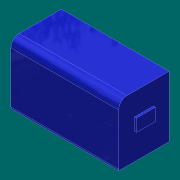
# Autodesk Inventor part: Blue tool box
Saved by Autodesk Inventor 2017 (Build 210142000, 142)
## iProperties
Created: 2018-01-23
Part Number: Blue tool box
Material: Steel
Document SubType Name: Modeling
Designer: Graeme_Van_Dongen
Density: 7.85 g/cm^3
Appearance: Blue - Wall Paint - Glossy
Author: Graeme_Van_Dongen
Autodesk Inventor part; units mm, degrees
ref_plane "YZ Plane" through (0, 0, 0) normal (1, 0, 0) x (0, 1, 0)
ref_plane "XZ Plane" through (0, 0, 0) normal (0, 1, 0) x (-1, 0, 0)
ref_plane "XY Plane" through (0, 0, 0) normal (0, 0, 1) x (1, 0, 0)
sketch "Sketch1" plane through (0, 0, 0) normal (0, 1, 0) x (-1, 0, 0)
  line L0 (330.2, 153.9875) -> (-330.2, 153.9875)
  line L1 (-330.2, 153.9875) -> (-330.2, -153.9875)
  line L2 (-330.2, -153.9875) -> (330.2, -153.9875)
  line L3 (330.2, -153.9875) -> (330.2, 153.9875)
  line L4 (330.2, 153.9875) -> (-330.2, -153.9875) construction
  line L5 (-330.2, 153.9875) -> (330.2, -153.9875) construction
  point P0 (0, 0)
  dimension "d0" = 660.4
  dimension "d1" = 307.975
  constraints: 12 end point, 2 midpoint, 2 parallel, 1 horizontal, 1 perpendicular
  measures "d0" distance of L2.end L1.end
  measures "d1" distance of L1.end L0.end
extrude "Extrusion1" add sketch "Sketch1" along normal blind 374.65
sketch "Sketch4" plane through (330.2, 0, 153.9875) normal (1, 0, 0) x (0, 0, -1)
  line L0 (96.8375, 161.925) -> (211.1375, 161.925)
  line L1 (211.1375, 161.925) -> (211.1375, 238.125)
  line L2 (211.1375, 238.125) -> (96.8375, 238.125)
  line L3 (96.8375, 238.125) -> (96.8375, 161.925)
  point P0 (153.9875, 0)
  point P1 (153.9875, 161.925)
  dimension "d11" = 114.3
  dimension "d12" = 161.925
  dimension "d13" = 76.2
  constraints: 8 end point, 2 parallel, 1 horizontal, 1 midpoint, 1 perpendicular, 1 vertical alignment
  measures "d11" distance of L2.end L1.end
  measures "d12" distance from line of point (153.987, 0) L0
  measures "d13" distance of L0.end L1.end
extrude "Extrusion4" add sketch "Sketch4" along normal blind 12.7
mirror "Mirror1" about plane through (0, 0, 0) normal (1, 0, 0) of "Extrusion4"
sketch "Sketch6" plane through (-330.2, 0, 153.9875) normal (0, 0, 1) x (1, 0, 0)
  line L0 (0, 374.65) -> (660.4, 374.65) projected
  line L1 (0, 374.65) -> (0, 9.525)
  line L2 (0, 9.525) -> (660.4, 9.525)
  line L3 (660.4, 9.525) -> (660.4, 374.65)
  point P0 (330.2, 0)
  dimension "d22" = 9.525
  constraints: 6 end point, 2 perpendicular, 1 vertical
  measures "d22" distance from line of point (330.2, 0) L2
extrude "Extrusion6" add sketch "Sketch6" along normal blind 1.5875
fillet "Fillet1" radius 50.8 1 edges at (0, 374.65, 155.575)
body "Solid1"
